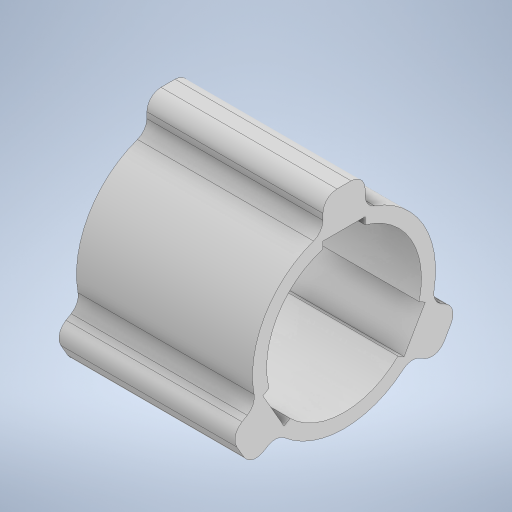
# Autodesk Inventor part: Part1
Saved by Autodesk Inventor 2024 (Build 280153000, 153)
## iProperties
Created: 2023-11-27
Part Number: Part1
Material: Generic
Document SubType Name: Modeling
Designer: kubad
Density: 1 g/cm^3
Appearance: Default
Author: kubad
Autodesk Inventor part; units mm, degrees
ref_plane "YZ Plane" through (0, 0, 0) normal (1, 0, 0) x (0, 1, 0)
ref_plane "XZ Plane" through (0, 0, 0) normal (0, 1, 0) x (-1, 0, 0)
ref_plane "XY Plane" through (0, 0, 0) normal (0, 0, 1) x (1, 0, 0)
sketch "Sketch1" plane through (0, 0, 0) normal (1, 0, 0) x (0, 1, 0)
  point P0 (0, 0)
sketch "Sketch2" plane through (0, 0, 0) normal (1, 0, 0) x (0, 1, 0)
  circle A0 centre (0, 0) radius 11
  circle A1 centre (0, 0) radius 13
  line L0 (0, 0) -> (13, 0)
  line L1 (0, 0) -> (-6.5, -11.2583)
  line L2 (0, 0) -> (13, 0) construction
  line L3 (0, 0) -> (-6.5, 11.2583)
  line L4 (0, 0) -> (13, 0) construction
  line L5 (11, 0) -> (11, -3)
  line L6 (11, 0) -> (11, 3)
  line L7 (-5.5, 9.5263) -> (-8.0981, 8.0263)
  line L8 (-5.5, 9.5263) -> (-2.9019, 11.0263)
  line L9 (-5.5, -9.5263) -> (-2.9019, -11.0263)
  line L10 (-5.5, -9.5263) -> (-8.0981, -8.0263)
  line L11 (11, 3) -> (15, 3)
  line L12 (15, 3) -> (11, 3)
  line L13 (11, 3) -> (11, -3)
  line L14 (11, -3) -> (15, -3)
  line L15 (15, -3) -> (15, 3)
  line L16 (-2.9019, 11.0263) -> (-4.9019, 14.4904)
  line L17 (-8.0981, 8.0263) -> (-10.0981, 11.4904)
  line L18 (-10.0981, 11.4904) -> (-4.9019, 14.4904)
  line L19 (-2.9019, -11.0263) -> (-4.9019, -14.4904)
  line L20 (-8.0981, -8.0263) -> (-10.0981, -11.4904)
  line L21 (-4.9019, -14.4904) -> (-10.0981, -11.4904)
  line L22 (-2.9019, 11.0263) -> (-2.6934, 10.6652)
  line L23 (-8.0981, 8.0263) -> (-7.8896, 7.6652)
  line L24 (-2.6934, 10.6652) -> (-3.1934, 11.5312)
  line L25 (-3.1934, 11.5312) -> (-8.3896, 8.5312)
  line L26 (-2.9019, -11.0263) -> (-2.6934, -10.6652)
  line L27 (-8.0981, -8.0263) -> (-7.8896, -7.6652)
  line L28 (-2.6934, -10.6652) -> (-3.1934, -11.5312)
  line L29 (-3.1934, -11.5312) -> (-8.3896, -8.5312)
  line L30 (11, -3) -> (10.583, -3)
  line L31 (11, 3) -> (10.583, 3)
  line L32 (10.583, -3) -> (11.583, -3)
  line L33 (11.583, -3) -> (11.583, 3)
  point P0 (-8.9226, 9.4545)
  point P1 (-8.9226, -9.4545)
  point P2 (-3.7265, -12.4545)
  point P3 (12.6491, -3)
  point P4 (12.6491, 3)
  point P5 (-3.7265, 12.4545)
  dimension "d0" = 22
  dimension "d1" = 26
  dimension "d2" = 120
  dimension "d3" = 120
  dimension "d4" = 3
  dimension "d5" = 3
  dimension "d6" = 3
  dimension "d7" = 3
  dimension "d8" = 3
  dimension "d9" = 3
  dimension "d10" = 4
  dimension "d11" = 4
  dimension "d12" = 4
  dimension "d13" = 4
  dimension "d14" = 4
  dimension "d15" = 1
  dimension "d16" = 1
  dimension "d17" = 1
  constraints: 68 end point, 9 perpendicular, 9 point on line, 5 horizontal, 4 parallel, 3 point on circle, 2 coincident, 2 equal length, 1 centre point, 1 vertical, 15 other
  measures "d1" diameter of A1
  measures "d2" angle of L1 L2
  measures "d3" angle of L4 L3
  measures "d4" distance of L5.start L5.end
  measures "d5" distance of L5.start L6.end
  measures "d6" distance of L7.start L7.end
  measures "d7" distance of L7.start L8.end
  measures "d8" distance of L9.start L9.end
  measures "d9" distance of L9.start L10.end
  measures "d10" distance of L6.end L11.end
  measures "d11" distance of L8.end L16.end
  measures "d12" distance of L7.end L17.end
  measures "d13" distance of L9.end L19.end
  measures "d14" distance of L10.end L20.end
  measures "d15" distance of L22.end L24.end
  measures "d16" distance of L26.end L28.end
  measures "d17" distance of L30.end L32.end
extrude "Extrusion1" add sketch "Sketch2" along normal blind 25 contours A0 L22 L16 A1 L11 L31 | L30 L14 A1 L19 L26 A0 | L33 L11 A1 L0 | L0 A1 L14 L33 | A1 L11 L15 L14 | L27 L20 A1 L17 L23 A0 | L29 L19 A1 L1 | L1 A1 L20 L29 | L25 L17 A1 L3 | L3 A1 L16 L25 | A1 L19 L21 L20 | A1 L17 L18 L16
sketch "Sketch3" plane through (25, 0, 0) normal (1, 0, 0) x (0, 0, -1)
  line L0 (3, 15) -> (-3, 15) projected
  line L1 (-3, 15) -> (3, 15)
  line L2 (3, 15) -> (3, 16.9996)
  line L3 (3, 16.9996) -> (-3, 16.9996)
  line L4 (-3, 16.9996) -> (-3, 15)
  line L5 (9.4545, -8.9226) -> (11.4904, -10.0981) projected
  line L6 (11.4904, -10.0981) -> (13.2224, -11.0981)
  line L7 (13.2224, -11.0981) -> (16.2224, -5.9019)
  line L8 (16.2224, -5.9019) -> (14.4904, -4.9019)
  line L9 (-11.4904, -10.0981) -> (-9.4545, -8.9226) projected
  line L10 (-11.4904, -10.0981) -> (-13.2224, -11.0981)
  line L11 (-13.2224, -11.0981) -> (-16.2224, -5.9019)
  line L12 (-14.4904, -4.9019) -> (-11.4904, -10.0981) projected
  line L13 (-16.2224, -5.9019) -> (-14.4904, -4.9019)
  point P0 (0, 0)
  dimension "d20" = 2
  dimension "d21" = 6
  dimension "d22" = 2
  dimension "d23" = 6
  constraints: 20 end point, 4 perpendicular, 2 collinear, 2 parallel, 1 horizontal
  measures "d20" distance of L5.end L6.end
  measures "d21" distance of L6.end L7.end
  measures "d22" distance of L9.start L10.end
  measures "d23" distance of L10.end L11.end
extrude "Extrusion2" add sketch "Sketch3" against normal blind 25 contours L0 L4 L3 L2
extrude "Extrusion3" add sketch "Sketch3" against normal blind 25 contours L10 L11 L13 L12
sketch "Sketch4" plane through (0, 0, 0) normal (-1, 0, 0) x (0, 0, 1)
  line L0 (-11.4904, -10.0981) -> (-14.4904, -4.9019) projected
  line L1 (-11.4904, -10.0981) -> (-14.4904, -4.9019)
  line L2 (-14.4904, -4.9019) -> (-16.2224, -5.9019)
  line L3 (-16.2224, -5.9019) -> (-13.2224, -11.0981)
  line L4 (-13.2224, -11.0981) -> (-11.4904, -10.0981)
  point P0 (0, 0)
  dimension "d28" = 2
  dimension "d29" = 6
  constraints: 8 end point, 2 perpendicular, 1 collinear
  measures "d28" distance of L0.end L2.end
  measures "d29" distance of L2.end L3.end
extrude "Extrusion4" add sketch "Sketch4" against normal blind 25
fillet "Fillet1" radius 2 12 edges at (12.5, -8.9226, -9.4545) (12.5, -11.0981, -13.2224) (12.5, -3.7265, -12.4545) (12.5, -5.9019, -16.2224) (12.5, 12.6491, -3) (12.5, 16.9996, -3) (12.5, 12.6491, 3) (12.5, 16.9996, 3) (12.5, -3.7265, 12.4545) (12.5, -5.9019, 16.2224) (12.5, -8.9226, 9.4545) (12.5, -11.0981, 13.2224)
body "Solid1"
